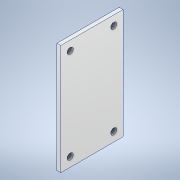
# Autodesk Inventor part: arm to water block plate
Saved by Autodesk Inventor 2021 (Build 250183000, 183)
## iProperties
Created: 2021-03-29
Part Number: arm to water block plate
Material: Aluminum 6061
Document SubType Name: Modeling
Designer: Work
Mass: 38.4673 g
Surface Area: 100.664 cm^2
Volume: 14.2471 cm^3
Density: 2.7 g/cm^3
Appearance: Aluminum - Flat
Author: Work
Autodesk Inventor part; units mm, degrees
ref_plane "YZ Plane" through (0, 0, 0) normal (1, 0, 0) x (0, 1, 0)
ref_plane "XZ Plane" through (0, 0, 0) normal (0, 1, 0) x (-1, 0, 0)
ref_plane "XY Plane" through (0, 0, 0) normal (0, 0, 1) x (1, 0, 0)
sketch "Sketch1" plane through (0, 0, 0) normal (1, 0, 0) x (0, 1, 0)
  line L0 (0, 0) -> (89.8652, 0)
  line L1 (89.8652, 0) -> (89.8652, -50.8)
  line L2 (89.8652, -50.8) -> (0, -50.8)
  line L3 (0, -50.8) -> (0, 0)
  dimension "d0" = 89.8652
  dimension "d1" = 50.8
  constraints: 8 end point, 2 parallel, 1 horizontal, 1 perpendicular
  measures "d0" distance of L1.end L2.end
  measures "d1" distance of L0.end L1.end
extrude "Extrusion1" add sketch "Sketch1" along normal blind 3.175
sketch "Sketch2" plane through (3.175, 0, 0) normal (1, 0, 0) x (0, 0, -1)
  line L0 (0, 89.8652) -> (0, 0) projected
  line L1 (50.8, 89.8652) -> (0, 89.8652) projected
  point P0 (7.62, 82.2452)
  dimension "d4" = 7.62
  dimension "d5" = 7.62
  measures "d4" distance from line of L0 point (7.62, 82.245)
  measures "d5" distance from line of L1 point (7.62, 82.245)
hole "Hole1" at (3.175, 82.2452, -7.62) direction (-1, 0, 0) diameter 4.9784 end through all
pattern_linear "Rectangular Pattern1" count 2 spacing 74.6252 along (0, -1, 0) count 2 spacing 35.56 along (0, 0, -1) of "Hole1"
body "Solid1"
